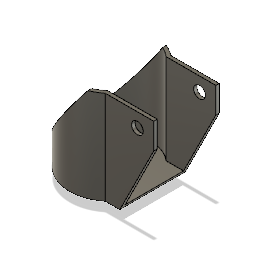
20part (Autodesk Fusion 360 design; units mm, degrees)
Autodesk Fusion 360 part; units mm, degrees
sketch "Sketch1" plane through (0, 0, 0) normal (0, 1, 0) x (1, 0, 0)
  line L0 (11.3137, 14) -> (32, 14)
  line L1 (32, 14) -> (32, -14)
  line L2 (32, -14) -> (11.3137, -14)
  arc A0 (11.3137, 14) -> (11.3137, -14) centre (0, 0) ccw
  line L3 (32, -12.5) -> (10.7703, -12.5)
  arc A1 (10.7703, 12.5) -> (10.7703, -12.5) centre (0, 0) ccw
  line L4 (10.7703, 12.5) -> (32, 12.5)
  circle A2 centre (0, 0) radius 2.75
  dimension "d1" = 36
  dimension "d4" = 1.5
  dimension "d5" = 5.5
  constraint coincident A0.centre A1.centre
  constraint horizontal L0
  constraint vertical L1
  constraint horizontal L2
  constraint concentric A0 A2
  measures "d1" diameter of A0
  measures "d5" diameter of A2
extrude "Extrude1" add sketch "Sketch1" along normal blind 40 contours L0 L1 L2 A0 L3 A1 L4 | L1 L3 A1 L4 | A2
extrude "Extrude2" cut sketch "Sketch1" along normal through all from surface at 1.5 contours L1 L3 A1 L4 | A2
extrude "Extrude3" add sketch "Sketch1" against normal blind 4 contours A2
sketch "Sketch2" plane through (0, 0, 0) normal (0, 0, 1) x (1, 0, 0)
  line L0 (15.3745, -4.2511) -> (35, 35)
  line L1 (35, 35) -> (35, 42)
  line L2 (35, 42) -> (8, 42)
  line L3 (8, 42) -> (-19, 5)
  line L4 (-19, 5) -> (-19, -4.2511)
  line L5 (-19, -4.2511) -> (15.3745, -4.2511)
  circle A0 centre (25, 34) radius 2.5
  dimension "d12" = 5
  constraint vertical L1
  constraint perpendicular L1 L2
  constraint perpendicular L2 L4
  constraint horizontal L5
  measures "d12" diameter of A0
extrude "Extrude4" cut sketch "Sketch2" along normal through all and the other way through all keep common part
